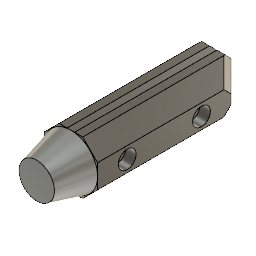
Hinge_Bracket_x2 (Autodesk Fusion 360 design; units mm, degrees)
Autodesk Fusion 360 part; units mm, degrees
sketch "Skizze1" plane through (0, 0, 0) normal (0, 0, 1) x (1, 0, 0)
  line L0 (0, 0) -> (12, 0)
  line L1 (6, 0) -> (6, 11.5)
  line L2 (6, 11.5) -> (15, 11.5)
  line L3 (6, 11.5) -> (-3, 11.5)
  line L4 (-3, 11.5) -> (0, 0)
  line L5 (12, 0) -> (15, 11.5)
  line L6 (6, 11.5) -> (7.25, 11.5)
  line L7 (6, 11.5) -> (4.75, 11.5)
  line L8 (7.25, 11.5) -> (15, 11.5)
  line L9 (15, 11.5) -> (15, 61.5)
  line L10 (15, 61.5) -> (7.25, 61.5)
  line L11 (7.25, 61.5) -> (7.25, 11.5)
  line L12 (4.75, 11.5) -> (-3, 11.5)
  line L13 (-3, 11.5) -> (-3, 61.5)
  line L14 (-3, 61.5) -> (4.75, 61.5)
  line L15 (4.75, 61.5) -> (4.75, 11.5)
  dimension "d1" = 12
  dimension "d2" = 11.5
  dimension "d3" = 9
  dimension "d4" = 9
  dimension "d5" = 1.25
  dimension "d6" = 1.25
  dimension "d7" = 50
  dimension "d8" = 50
  constraint coincident L0.start L4.end
  constraint horizontal L0
  constraint midpoint L0 L1.start
  constraint perpendicular L0 L1
  constraint perpendicular L1 L2
  constraint perpendicular L1 L3
  constraint perpendicular L1 L6
  constraint perpendicular L1 L7
  constraint horizontal L8
  constraint vertical L9
  constraint horizontal L10
  constraint vertical L11
  constraint horizontal L12
  constraint vertical L13
  constraint horizontal L14
  constraint vertical L15
  measures "d1" distance of L0.start L0.end
  measures "d2" distance of L1.start L1.end
  measures "d3" distance of L1.end L2.end
  measures "d4" distance of L1.end L3.end
  measures "d5" distance of L1.end L6.end
  measures "d6" distance of L1.end L7.end
  measures "d7" distance of L6.end L10.end
  measures "d8" distance of L7.end L14.end
  measures "d17" distance of L0.end
  measures "d30" distance of L0.end
revolve "Drehen1" add sketch "Skizze1" angle 360 about axis through (6, 0, 0) along (0, 1, 0) contours L0 L1 L3 L4 L7 L12
extrude "Extrusion1" add sketch "Skizze1" along normal blind 9 contours L3 L12 L13 L14 L15 | L2 L8 L9 L10 L11
extrude "Extrusion2" add sketch "Skizze1" against normal blind 9 contours L3 L12 L13 L14 L15 | L2 L8 L9 L10 L11
chamfer "Fase1" distance 5 angle 45 6 edges at (-3, 61.5, 0) (-3, 36.5, 9) (-3, 36.5, -9) (15, 36.5, 9) (15, 36.5, -9) (15, 61.5, 0)
sketch "Skizze2" plane through (15, 0, 0) normal (1, 0, 0) x (0, 1, 0)
  line L0 (56.5, 4) -> (11.5, 4)
  line L1 (11.5, 4) -> (11.5, 0)
  line L2 (11.5, 0) -> (11.5, -4)
  line L3 (11.5, -4) -> (56.5, -4)
  line L4 (56.5, -4) -> (56.5, 4)
  line L5 (11.5, 0) -> (21.5, 0)
  line L6 (56.5, 0) -> (46.5, 0)
  dimension "d15" = 10
  dimension "d16" = 10
  constraint coincident L1.end L2.start
  constraint perpendicular L1 L5
  constraint midpoint L4 L6.start
  constraint perpendicular L4 L6
  measures "d15" distance of L1.end L5.end
  measures "d16" distance of L6.start L6.end
sketch "Skizze3" plane through (-3, 0, 0) normal (-1, 0, 0) x (0, -1, 0)
  line L0 (-56.5, -4) -> (-11.5, -4)
  line L1 (-11.5, -4) -> (-11.5, 0)
  line L2 (-11.5, 0) -> (-11.5, 4)
  line L3 (-11.5, 4) -> (-56.5, 4)
  line L4 (-56.5, 4) -> (-56.5, -4)
  line L5 (-11.5, 0) -> (-21.5, 0)
  line L6 (-56.5, 0) -> (-46.5, 0)
  line L7 (-48.1454, 2.85) -> (-49.7909, 0)
  line L8 (-49.7909, 0) -> (-48.1454, -2.85)
  line L9 (-48.1454, -2.85) -> (-44.8546, -2.85)
  line L10 (-44.8546, -2.85) -> (-43.2091, 0)
  line L11 (-43.2091, 0) -> (-44.8546, 2.85)
  line L12 (-44.8546, 2.85) -> (-48.1454, 2.85)
  line L13 (-23.1454, 2.85) -> (-24.7909, 0)
  line L14 (-24.7909, 0) -> (-23.1454, -2.85)
  line L15 (-23.1454, -2.85) -> (-19.8546, -2.85)
  line L16 (-19.8546, -2.85) -> (-18.2091, 0)
  line L17 (-18.2091, 0) -> (-19.8546, 2.85)
  line L18 (-19.8546, 2.85) -> (-23.1454, 2.85)
  point P0 (-56.5, 0)
  point P1 (-46.5, 0)
  point P2 (-21.5, 0)
  dimension "d17" = 10
  dimension "d18" = 10
  dimension "d29" = 2.85
  dimension "d30" = 2.85
  constraint coincident L1.end L2.start
  constraint perpendicular L2 L5
  constraint coincident P0 L6.start
  constraint perpendicular L4 L6
  constraint coincident P1 L6.end
  constraint coincident P2 L5.end
  measures "d17" distance of L1.end P2
  measures "d18" distance of P0 P1
  measures "d29" distance of P1 L12
  measures "d30" distance of P2 L18
hole "Bohrung1" at (15, 46.5, 0) direction (-1, 0, 0) diameter 3.6 depth 25 tip angle 180 counterbore diameter 6 counterbore depth 3.5
hole "Bohrung2" at (15, 21.5, 0) direction (-1, 0, 0) diameter 3.6 depth 25 tip angle 180 counterbore diameter 6 counterbore depth 3.5
extrude "Extrusion3" cut sketch "Skizze3" against normal blind 2.6 contours L7 L8 L9 L10 L11 L12 | L13 L14 L15 L16 L17 L18
chamfer "Fase2" distance 2 angle 45 8 edges at (8.625, 61.5, 9) (12.5, 59, 6.5) (12.5, 59, -6.5) (8.625, 61.5, -9) (-0.5, 59, -6.5) (3.375, 61.5, -9) (-0.5, 59, 6.5) (3.375, 61.5, 9)
